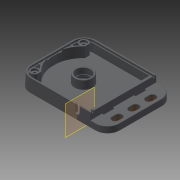
# Autodesk Inventor part: 276-2156
Saved by Autodesk Inventor 2016 SP2 (Build 200236200, 236)
## iProperties
Category: Sensors
Company: Autodesk Inc.
Created: 2012-04-02
Part Number: 276-2156
Document SubType Name: Modeling
Designer: Autodesk Inc.
Density: 1.42 g/cm^3
Material: Acetal Resin, White
Catalog Web Link: http://www.vexrobotics.com/276-2156.html
Vendor: VEX
Mass: 13.8512 g
Surface Area: 116.5 cm^2
Volume: 9.75434 cm^3
Appearance: Gray
Author: Autodesk Inc.
Autodesk Inventor part; units mm, degrees
(part 1 of 3)
sketch "Sketch1" plane through (0, 0, 0) normal (0, 0, 1) x (1, 0, 0)
  line L0 (61.4848, -6.4998) -> (61.4848, 43.5002)
  line L1 (53.0765, 43.5002) -> (-6.0152, 43.5002)
  line L2 (-6.0152, 43.5002) -> (-6.0152, -6.4998)
  line L3 (-6.0152, 43.5002) -> (61.4848, 43.5002)
  line L4 (-6.0152, -6.4998) -> (61.4848, -6.4998)
  constraints: 10 end point, 1 parallel
extrude "Extrusion1" add sketch "Sketch1" against normal blind 9.4996 draft -2
ref_plane "Work Plane1" through (-6.0152, -6.4998, 0) normal (0, 1, 0) x (1, 0, 0)
sketch "Sketch2" plane through (-6.0152, -6.4998, 0) normal (0, 1, 0) x (1, 0, 0)
  line L0 (0.3317, 9.4996) -> (67.1683, 9.4996)
  line L1 (67.5, 0) -> (67.1683, 9.4996)
  line L2 (0, 0) -> (67.5, 0)
  line L3 (0, 0) -> (0.3317, 9.4996)
  line L4 (0.157, 4.4958) -> (13.081, 4.4958)
  line L5 (13.081, 4.4958) -> (13.1683, 9.4996)
  point P0 (6.0152, 0)
  dimension "d3" = 5.0038
  dimension "d4" = 91
  dimension "d5" = 13.081
  constraints: 4 end point, 2 point on line, 1 parallel
  measures "d3" distance between parallel lines of L0 L4
  measures "d4" angle of L5 L4
  measures "d5" horizontal distance of L4.end L2.start
extrude "Extrusion2" cut sketch "Sketch2" along normal up to next contours L0 L5 L4 L3
fillet "Fillet1" radius 8.9916 4 edges at (61.3189, -6.3339, -4.7498) (-5.9367, -6.4213, -2.2479) (-5.9367, 43.4217, -2.2479) (61.3189, 43.3344, -4.7498)
ref_plane "Work Plane2" through (0, 0, -8.001) normal (0, 0, -1) x (-1, 0, 0)
sketch "Sketch5" plane through (0, 0, -9.4996) normal (0, 0, -1) x (-1, 0, 0)
  line L0 (-7.1531, -6.168) -> (-7.1531, 43.1685)
  line L1 (-52.1669, 43.1685) -> (-7.1531, 43.1685)
  arc A0 (-60.1554, 2.5074) -> (-52.4976, -5.1612) centre (-52.4864, 2.5078) ccw
  line L2 (-60.1554, 2.5074) -> (-60.1554, 34.509)
  arc A1 (-52.4904, 42.1754) -> (-60.1554, 34.509) centre (-52.4891, 34.509) ccw
  line L3 (-52.4904, 42.1754) -> (-7.6488, 42.1754)
  line L4 (-7.6488, 43.1685) -> (-52.4917, 43.1685)
  arc A2 (-52.4917, 43.1685) -> (-61.1599, 34.5002) centre (-52.4917, 34.5002) ccw
  line L5 (-18.6416, -6.168) -> (-52.4917, -6.168)
  ellipse E0 centre (-18.6417, -5.8678) end of major axis (-18.5647, -6.158) minor radius 0.3 (-18.6416, -6.168) -> (-18.3417, -5.8679) ccw
  line L6 (-18.3417, -5.8679) -> (-18.3417, -5.1612)
  line L7 (-7.1313, -5.1612) -> (-52.4976, -5.1612)
  arc A3 (-59.5458, 2.5026) -> (-52.4917, -4.5516) centre (-52.4917, 2.5026) ccw
  line L8 (-59.5458, 2.5026) -> (-59.5458, 5.6742)
  line L9 (-59.5458, 2.5026) -> (-59.5458, 34.5071)
  arc A4 (-52.4917, 41.5612) -> (-59.5458, 34.5071) centre (-52.4917, 34.5071) ccw
  line L10 (-8.9376, 41.5612) -> (-8.9376, -3.8612)
  line L11 (-8.9376, 40.8754) -> (-7.1313, 40.8754)
  line L12 (-7.1313, 40.8754) -> (-7.1313, 42.1832)
  line L13 (-7.1313, 42.1832) -> (-52.4904, 42.1754)
  arc A5 (-52.4904, 42.1754) -> (-60.1586, 34.5071) centre (-52.4904, 34.5071) ccw
  line L14 (-60.1586, 34.5071) -> (-60.1599, 2.5071)
  arc A6 (-60.1599, 2.5071) -> (-52.4917, -5.1612) centre (-52.4917, 2.5071) ccw
  line L15 (-52.4917, -5.1612) -> (-18.3278, -5.1612)
  line L16 (-8.9376, -4.5516) -> (-52.4917, -4.5516)
  line L17 (-8.9376, -3.8612) -> (-8.9376, -4.5516)
  line L18 (-8.9376, -3.8612) -> (-7.1313, -3.8612)
  line L19 (-7.1313, -3.8612) -> (-7.1313, -5.1612)
  line L20 (-52.4917, 41.5612) -> (-8.9376, 41.5612)
  line L21 (-7.1531, -6.168) -> (-52.1669, -6.168)
  line L22 (-8.9376, 41.5612) -> (-52.4917, 41.5612)
  arc A7 (-52.4917, 41.5612) -> (-59.5458, 34.5071) centre (-52.4917, 34.5071) ccw
  line L23 (-59.5458, 34.5071) -> (-59.5458, 2.5026)
  arc A8 (-59.5458, 2.5026) -> (-52.4917, -4.5516) centre (-52.4917, 2.5026) ccw
  line L24 (-52.4917, -4.5516) -> (-8.9376, -4.5516)
  line L25 (-8.9376, -4.5516) -> (-8.9376, 41.5612)
  point P0 (0, 0)
  point P1 (-6.9917, 18.5071)
  point P2 (-52.4917, 34.5071)
  dimension "d10" = 8.6614
  dimension "d13" = 0.9931
  dimension "d14" = 0.6096
  dimension "d15" = 0.6096
  dimension "d16" = 7.0541
  dimension "d17" = 7.6682
  dimension "d18" = 8.6683
  dimension "d19" = 7.0541
  constraints: 46 end point, 20 point on circle, 14 tangent, 9 centre point, 6 collinear, 5 perpendicular, 3 parallel, 3 vertical, 2 horizontal, 2 point on line, 5 other
  measures "d10" distance from line of point (-52.492, 34.507) L1
  measures "d13" distance between parallel lines of L3 L4
  measures "d14" distance between parallel lines of L16 L15
  measures "d15" distance between parallel lines of L2 L9
  measures "d16" radius of A4
  measures "d17" radius of A5
  measures "d18" radius of A2
  measures "d19" radius of A3
extrude "Extrusion3" cut sketch "Sketch5" against normal blind 1.4986 contours L7 A0 L2 A1 L13 L0 L11 L10 L20 A4 L9 L8 A3 L16 L17 L18 | L0 L18 L19 L7 | L0 L13 L12 L11 | L17 L16 A3 L8 L9 A4 L20 L10
extrude "Extrusion4" cut sketch "Sketch5" against normal blind 6.1976 draft -0.5 contours L17 L16 A3 L8 L9 A4 L20 L10
sketch "Sketch9" plane through (0, 0, 0) normal (0, 0, 1) x (1, 0, 0)
  circle A0 centre (37.0754, 18.4938) radius 4.7498
  circle A1 centre (37.0754, 18.4938) radius 5.3086
  point P0 (0, 0)
  dimension "d36" = 10.6172
  constraints: 1 centre point, 1 coincident
  measures "d36" diameter of A1
sketch "Sketch10" plane through (0, 0, -9.4996) normal (0, 0, -1) x (-1, 0, 0)
  circle A0 centre (-37.0754, 18.4938) radius 4.7498
  arc A1 (-56.912, 5.8938) -> (-52.4754, 0.7431) centre (-37.0754, 18.4938) ccw
  line L0 (-52.4754, 0.7431) -> (-52.4754, 1.9978)
  arc A2 (-59.5458, 16.4056) -> (-52.4754, 1.9978) centre (-37.0754, 18.4938) ccw
  line L1 (-58.9436, 12.9209) -> (-58.9436, 9.8898)
  arc A3 (-60.1436, 14.0099) -> (-57.6251, 7.0938) centre (-37.0754, 18.4938) ccw
  line L2 (-57.6251, 7.0938) -> (-60.1436, 7.0938)
  line L3 (-58.9436, 7.0938) -> (-58.9436, 5.8938)
  line L4 (-60.1436, 5.8938) -> (-56.912, 5.8938)
  line L5 (-58.9436, 7.0938) -> (-57.6251, 7.0938)
  arc A4 (-58.9436, 9.8898) -> (-57.6251, 7.0938) centre (-37.0754, 18.4938) ccw
  line L6 (-58.9436, 9.8898) -> (-58.9436, 12.9209)
  arc A5 (-58.9436, 12.9209) -> (-52.4754, 1.9978) centre (-37.0754, 18.4938) ccw
  line L7 (-52.4754, 1.9978) -> (-52.4754, 0.7431)
  arc A6 (-56.912, 5.8938) -> (-52.4754, 0.7431) centre (-37.0754, 18.4938) ccw
  line L8 (-56.912, 5.8938) -> (-58.9436, 5.8938)
  line L9 (-58.9436, 5.8938) -> (-58.9436, 7.0938)
  line L10 (-57.6251, 29.8938) -> (-60.1436, 29.8938)
  line L11 (-58.9436, 29.8938) -> (-58.9436, 31.0938)
  line L12 (-60.1436, 31.0938) -> (-56.912, 31.0938)
  arc A7 (-52.4754, 36.2446) -> (-56.912, 31.0938) centre (-37.0754, 18.4938) ccw
  line L13 (-52.4754, 36.2446) -> (-52.4754, 34.9898)
  arc A8 (-52.4754, 34.9898) -> (-59.5458, 20.5821) centre (-37.0754, 18.4938) ccw
  line L14 (-58.9436, 24.0668) -> (-58.9436, 27.0979)
  arc A9 (-57.6251, 29.8938) -> (-60.1436, 22.9778) centre (-37.0754, 18.4938) ccw
  arc A10 (-52.4754, 42.1621) -> (-60.1436, 34.4938) centre (-52.4754, 34.4938) ccw
  line L15 (-60.1436, 34.4938) -> (-60.1436, 2.4938)
  arc A11 (-60.1436, 2.4938) -> (-52.4754, -5.1744) centre (-52.4754, 2.4938) ccw
  arc A12 (-61.1436, 2.4938) -> (-52.4754, -6.1744) centre (-52.4754, 2.4938) ccw
  line L16 (-61.1436, 2.4938) -> (-61.1436, 34.4938)
  arc A13 (-52.4754, 43.1621) -> (-61.1436, 34.4938) centre (-52.4754, 34.4938) ccw
  arc A14 (-57.0545, -2.8468) -> (-52.4754, -1.2562) centre (-55.4754, -0.0062) ccw
  line L17 (-52.4754, -1.2562) -> (-52.4754, 0.7431)
  arc A15 (-54.9133, 3.1949) -> (-52.4754, 0.7431) centre (-37.0754, 18.4938) ccw
  arc A16 (-54.9133, 3.1949) -> (-58.5542, -1.0471) centre (-55.4754, -0.0062) ccw
  arc A17 (-58.5542, -1.0471) -> (-57.0545, -2.8468) centre (-52.4754, 2.4938) ccw
  circle A18 centre (-55.4754, -0.0062) radius 2.2762
  arc A19 (-52.4754, 36.2446) -> (-54.9133, 33.7928) centre (-37.0754, 18.4938) ccw
  line L18 (-52.4754, 36.2446) -> (-52.4754, 38.2438)
  arc A20 (-52.4754, 38.2438) -> (-57.0545, 39.8344) centre (-55.4754, 36.9938) ccw
  arc A21 (-57.0545, 39.8344) -> (-58.5542, 38.0348) centre (-52.4754, 34.4938) ccw
  arc A22 (-58.5542, 38.0348) -> (-54.9133, 33.7928) centre (-55.4754, 36.9938) ccw
  circle A23 centre (-55.4754, 36.9938) radius 2.2762
  line L19 (-59.5458, 2.5026) -> (-59.5458, 34.5071)
  point P0 (0, 0)
  constraints: 46 point on circle, 38 end point, 23 centre point, 12 point on line
extrude "Extrusion10" add sketch "Sketch10" against normal up to surface (6.1976 mm away) contours L4 L3 L2 A3 L1 A2 L0 A1 | L4 L19 L2 L3 | L4 L15 L2 L19 | L1 A3 L19 A2 | A3 L15 A9 L19 | L19 A9 L14 A8 | L14 A9 L10 L11 L12 A7 L13 A8 | L15 L12 L19 L10 | L19 L12 L11 L10
sketch "Sketch11" plane through (0, 0, -9.4996) normal (0, 0, -1) x (-1, 0, 0)
  line L0 (-60.1554, 2.5074) -> (-60.1554, 34.509)
  line L1 (-60.1554, 5.8904) -> (-60.1554, 7.1091)
  line L2 (-59.5458, 2.5026) -> (-59.5458, 34.5071)
  line L3 (-60.1436, 34.4938) -> (-60.1436, 2.4938)
  line L4 (-59.5458, 29.8998) -> (-60.1436, 29.8998)
  line L5 (-60.1436, 29.8998) -> (-60.1436, 31.0963)
  line L6 (-60.1436, 31.0963) -> (-59.5458, 31.0963)
  line L7 (-59.5458, 31.0963) -> (-59.5458, 29.8998)
  line L8 (-60.1436, 5.8938) -> (-56.912, 5.8938)
  line L9 (-59.5458, 5.8938) -> (-60.1436, 5.8938)
  line L10 (-60.1436, 5.8938) -> (-60.1436, 7.0942)
  line L11 (-60.1436, 7.0942) -> (-59.5458, 7.0942)
  line L12 (-59.5458, 7.0942) -> (-59.5458, 5.8938)
  line L13 (-58.9436, 9.8898) -> (-58.9436, 12.9209)
  arc A0 (-60.1436, 14.0099) -> (-57.6251, 7.0938) centre (-37.0754, 18.4938) ccw
  arc A1 (-57.6251, 29.8938) -> (-60.1436, 22.9778) centre (-37.0754, 18.4938) ccw
  line L14 (-58.9436, 24.0668) -> (-58.9436, 27.0979)
  arc A2 (-52.4754, 34.9898) -> (-59.5458, 20.5821) centre (-37.0754, 18.4938) ccw
  line L15 (-59.5458, 16.4056) -> (-59.5458, 20.5821)
  arc A3 (-59.5458, 16.4056) -> (-52.4754, 1.9978) centre (-37.0754, 18.4938) ccw
  point P0 (0, 0)
  constraints: 18 end point, 6 point on line, 4 parallel, 2 horizontal, 2 perpendicular
extrude "Extrusion11" cut sketch "Sketch11" against normal up to surface (1.4986 mm away) contours L8 L3 L11 L2 | A0 L3 A1 L2 | L2 A3 L13 A0 | L2 A1 L14 A2 | L3 L6 L2 L4
extrude "Extrusion12" add sketch "Sketch10" against normal up to surface (6.1976 mm away) contours A1 L17 A14 A17 A16 | A7 A22 A21 A20 L18 | A18 | A23
extrude "Extrusion13" cut sketch "Sketch10" against normal blind 1.4986 contours A18 | A23
hole "Hole1" at (55.4754, -0.0062, -9.4996) at (55.4754, 36.9938, -9.4996) direction (0, 0, 1) diameter 2.1082 end through all
ref_plane "Work Plane3" through (27.7348, -6.4998, 0) normal (0, 1, 0) x (-1, 0, 0)
sketch "Sketch12" plane through (27.7348, -6.4998, 0) normal (0, 1, 0) x (-1, 0, 0)
  line L0 (24.7639, 0) -> (-24.7639, 0)
  line L1 (9.4422, -3.81) -> (12.0584, -3.81)
  line L2 (12.0584, -3.81) -> (12.116, -9.4996)
  line L3 (9.4422, -3.81) -> (9.3846, -9.4996)
  line L4 (20.5817, -9.4996) -> (-24.4321, -9.4996)
  point P0 (27.7348, 0)
  point P1 (20.669, -4.4958)
  dimension "d59" = 3.81
  dimension "d60" = 8.6106
  dimension "d61" = 90.58
  dimension "d62" = 90.58
  dimension "d63" = 2.6162
  constraints: 6 end point, 2 point on line, 1 parallel
  measures "d59" distance between parallel lines of L1 L0
  measures "d60" horizontal distance of L1.end point (20.669, -4.496)
  measures "d61" angle of L2 L1
  measures "d62" angle of L3 L1
  measures "d63" distance of L1.start L1.end
extrude "Extrusion14" cut sketch "Sketch12" along normal up to next
fillet "Fillet6" radius 0.508 5 edges at (18.3214, -6.2674, -6.6548) (16.9845, -6.3667, -3.81) (15.6476, -6.2674, -6.6548) (18.2926, -5.4343, -3.81) (15.6764, -5.4343, -3.81)
extrude "Extrusion15" cut sketch "Sketch10" against normal up to surface (1.4986 mm away) contours L4 L19 L2 L3 | L4 L15 L2 L19 | L15 L12 L19 L10 | L19 L12 L11 L10
sketch "Sketch13" plane through (0, 0, 0) normal (0, 0, 1) x (1, 0, 0)
  line L0 (52.4987, 43.5002) -> (2.9709, 43.5002)
  line L1 (-6.0152, 34.5141) -> (-6.0152, 2.4864)
  line L2 (2.9709, -6.4998) -> (52.4987, -6.4998)
  point P0 (0, 0)
  point P1 (12.0442, 36.9978)
  point P2 (12.0442, 0.0026)
  dimension "d69" = 6.5024
  dimension "d70" = 18.0594
  dimension "d71" = 6.5024
  constraints: 1 vertical alignment
  measures "d69" distance from line of L0 point (12.044, 36.998)
  measures "d70" distance from line of L1 point (12.044, 36.998)
  measures "d71" distance from line of L2 point (12.044, 0.003)
hole "Hole2" at (12.0442, 36.9978, 0) at (12.0442, 0.0026, 0) direction (0, 0, -1) diameter 3.7846 depth 3.302
fillet "Fillet7" radius 0.508 2 edges at (12.0442, 1.8949, 0) (12.0442, 38.8901, 0)
sketch "Sketch14" plane through (7.0658, -6.3428, -4.4958) normal (0, 0, -1) x (-1, 0, 0)
  arc A0 (1.2904, 16.6628) -> (1.0904, 16.8628) centre (1.0904, 16.6628) ccw
  line L0 (1.2904, 16.6628) -> (1.2904, 9.0104)
  arc A1 (1.0904, 8.8104) -> (1.2904, 9.0104) centre (1.0904, 9.0104) ccw
  line L1 (1.0904, 8.8104) -> (0.2119, 8.8104)
  ellipse E0 centre (0.2119, 9.0104) end of major axis (0.3908, 9.0999) minor radius 0.2 (0.0119, 9.0104) -> (0.2119, 8.8104) ccw
  line L2 (3.9556, 0.4766) -> (0.0119, 0.4766)
  ellipse E1 centre (3.9461, 8.9809) end of major axis (-2.0703, 14.9981) minor radius 8.4995 (3.9556, 0.4766) -> (12.4504, 8.9714) ccw
  line L3 (12.4504, 40.7018) -> (12.4504, 8.9714)
  ellipse E2 centre (3.9461, 40.6923) end of major axis (9.9626, 46.7095) minor radius 8.4995 (12.4504, 40.7018) -> (3.9556, 49.1966) ccw
  ellipse E3 centre (0.2121, 40.6628) end of major axis (0.0332, 40.7522) minor radius 0.2 (0.2121, 40.8628) -> (0.0121, 40.6628) ccw
  line L4 (1.0907, 40.8628) -> (0.2121, 40.8628)
  arc A2 (1.2904, 40.6628) -> (1.0907, 40.8628) centre (1.0904, 40.6628) ccw
  line L5 (1.2904, 40.6628) -> (1.2904, 33.0104)
  arc A3 (1.0904, 32.8104) -> (1.2904, 33.0104) centre (1.0904, 33.0104) ccw
  line L6 (1.0904, 32.8104) -> (0.2119, 32.8104)
  ellipse E4 centre (0.2119, 33.0104) end of major axis (0.3908, 33.0999) minor radius 0.2 (0.0119, 33.0104) -> (0.2119, 32.8104) ccw
  ellipse E5 centre (0.2119, 16.6628) end of major axis (0.033, 16.7522) minor radius 0.2 (0.2119, 16.8628) -> (0.0119, 16.6628) ccw
  line L7 (1.0904, 16.8628) -> (0.2119, 16.8628)
  arc A4 (10.8404, 26.3366) -> (5.3404, 26.3366) centre (8.0904, 26.3366) ccw
  line L8 (10.8404, 23.3366) -> (10.8404, 26.3366)
  arc A5 (5.3404, 23.3366) -> (10.8404, 23.3366) centre (8.0904, 23.3366) ccw
  line L9 (5.3404, 26.3366) -> (5.3404, 23.3366)
  arc A6 (10.8404, 39.0366) -> (5.3404, 39.0366) centre (8.0904, 39.0366) ccw
  line L10 (10.8404, 36.0366) -> (10.8404, 39.0366)
  arc A7 (5.3404, 36.0366) -> (10.8404, 36.0366) centre (8.0904, 36.0366) ccw
  line L11 (5.3404, 39.0366) -> (5.3404, 36.0366)
  arc A8 (10.8404, 13.6366) -> (5.3404, 13.6366) centre (8.0904, 13.6366) ccw
  line L12 (10.8404, 10.6366) -> (10.8404, 13.6366)
  arc A9 (5.3404, 10.6366) -> (10.8404, 10.6366) centre (8.0904, 10.6366) ccw
  line L13 (5.3404, 13.6366) -> (5.3404, 10.6366)
  line L14 (0.0119, 9.0104) -> (0.0119, 16.6628)
  line L15 (0.0121, 33.0005) -> (0.0121, 40.6628)
  point P0 (7.0658, 6.3428)
  point P1 (0.0904, 24.8366)
  point P2 (-30.0215, 24.36)
  point P3 (-30.0096, 24.8366)
  constraints: 32 end point, 20 point on circle, 10 centre point, 2 parallel, 28 other
extrude "Extrusion17" cut sketch "Sketch14" against normal blind 2.9972 contours L0 A1 L1 E0 L14 E5 L7 A0 | L4 A2 L5 A3 L6 E4 L15 E3
sketch "Sketch18" plane through (0, 0, -3.302) normal (0, 0, -1) x (-1, 0, 0)
  circle A0 centre (-12.0442, 0.0026) radius 1.8923
  circle A1 centre (-12.0442, 36.9978) radius 1.8923
  arc A2 (-56.9239, -2.9155) -> (-52.4754, -1.2562) centre (-55.4754, -0.0062) ccw
  arc A3 (-56.9239, -2.9155) -> (-52.4917, -4.4975) centre (-52.4917, 2.5026) ccw
  line L0 (-52.4917, -4.4975) -> (-8.9916, -4.4975)
  line L1 (-8.9916, -4.4975) -> (-8.9916, 41.5071)
  line L2 (-8.9916, 41.5071) -> (-52.4917, 41.5071)
  arc A4 (-52.4917, 41.5071) -> (-56.9935, 39.8675) centre (-52.4917, 34.5071) ccw
  arc A5 (-52.4754, 38.2438) -> (-56.9935, 39.8675) centre (-55.4754, 36.9938) ccw
  line L3 (-52.4754, 38.2438) -> (-52.4754, 34.9898)
  arc A6 (-52.4754, 34.9898) -> (-59.4917, 21.0993) centre (-37.0754, 18.4938) ccw
  line L4 (-59.4917, 21.0993) -> (-59.4917, 15.8884)
  arc A7 (-59.4917, 15.8884) -> (-52.4754, 1.9978) centre (-37.0754, 18.4938) ccw
  line L5 (-52.4754, 1.9978) -> (-52.4754, -1.2562)
  circle A8 centre (-37.0754, 18.4938) radius 7.2429
  point P0 (0, 0)
extrude "Extrusion20" cut sketch "Sketch18" against normal blind 1.4986 contours A2 L5 A7 L4 A6 L3 A5 A4 L2 L1 L0 A3 | A8
sketch "Sketch19" plane through (0, 0, -1.8034) normal (0, 0, -1) x (-1, 0, 0)
  arc A0 (-59.4917, 15.8884) -> (-52.4754, 1.9978) centre (-37.0754, 18.4938) ccw
  circle A1 centre (-37.0754, 18.4938) radius 6.7437
  point P0 (-37.0754, 18.4938)
  point P1 (0, 0)
  dimension "d92" = 13.4874
  constraints: 1 centre point, 1 coincident
  measures "d92" diameter of A1
extrude "Extrusion21" add sketch "Sketch19" along normal blind 6.2484 draft -1
sketch "Sketch20" plane through (37.0754, 18.4938, -8.0518) normal (0, 0, -1) x (-1, 0, 0)
  circle A0 centre (0, 0) radius 6.6346
  circle A1 centre (0, 0) radius 5.2451
  point P0 (37.0754, -18.4938)
  dimension "d95" = 10.4902
  constraints: 1 centre point, 1 coincident
  measures "d95" diameter of A1
extrude "Extrusion22" cut sketch "Sketch20" against normal blind 4.5466 contours A1
sketch "Sketch21" plane through (37.0754, 18.4938, -3.5052) normal (0, 0, -1) x (-1, 0, 0)
  circle A0 centre (0, 0) radius 5.2451
  circle A1 centre (0, 0) radius 4.7498
  point P0 (37.0754, -18.4938)
  dimension "d98" = 9.4996
  constraints: 1 centre point, 1 coincident
  measures "d98" diameter of A1
extrude "Extrusion23" cut sketch "Sketch21" against normal through all contours A1
extrude "Extrusion24" cut sketch "Sketch9" against normal blind 2.159
fillet "Fillet10" radius 1.4986 1 edges at (31.7668, 18.4938, 0)
fillet "Fillet11" radius 0.508 2 edges at (31.7668, 18.4938, -2.159) (41.8252, 18.4938, -2.159)
fillet "Fillet12" radius 0.508 2 edges at (43.71, 18.4938, -8.0518) (42.3205, 18.4938, -8.0518)
sketch "Sketch22" plane through (0, 0, 0) normal (0, 0, 1) x (1, 0, 0)
  line L0 (-6.004, 2.4925) -> (-6.004, 34.5035)
  line L1 (-6.004, 34.5035) -> (-6.004, 2.4925)
  ellipse E0 centre (-4.7038, 16.343) end of major axis (-4.4914, 16.5554) minor radius 0.3 (-5.004, 16.3427) -> (-4.7042, 16.0429) ccw
  spline S0 degree 3 poles (-5.379, 16.1568) (-5.3713, 16.112) (-5.3586, 16.0685) (-5.3265, 15.991) (-5.3082, 15.9569) (-5.2649, 15.8923) (-5.2385, 15.8606) (-5.1846, 15.8064) (-5.155, 15.7821) (-5.0906, 15.7392) (-5.0541, 15.7199) (-4.9466, 15.6745) (-4.8699, 15.6592) (-4.7883, 15.6589) knots 0.106772 0.106772 0.106772 0.106772 0.25 0.25 0.375 0.375 0.5 0.5 0.625 0.625 0.75 0.75 1 1 1 1
  spline S1 degree 3 poles (-5.388, 16.2585) (-5.3876, 16.1781) (-5.3714, 16.0993) (-5.3265, 15.991) (-5.3082, 15.9569) (-5.2649, 15.8923) (-5.2385, 15.8606) (-5.1846, 15.8064) (-5.155, 15.7821) (-5.0906, 15.7392) (-5.0541, 15.7199) (-4.9466, 15.6745) (-4.8699, 15.6592) (-4.7883, 15.6589) knots 0 0 0 0 0.25 0.25 0.375 0.375 0.5 0.5 0.625 0.625 0.75 0.75 1 1 1 1
  spline S2 degree 3 poles (-5.388, 16.2585) (-5.3878, 16.2242) (-5.3848, 16.1901) (-5.379, 16.1568) knots 0 0 0 0 1 1 1 1
  spline S3 degree 3 poles (-5.379, 16.1568) (-5.3755, 16.1426) (-5.3722, 16.1319) (-5.3702, 16.1262) (-5.3698, 16.1252) (-5.3695, 16.1244) (-5.3694, 16.1244) (-5.3693, 16.124) (-5.3691, 16.1237) (-5.369, 16.1236) (-5.369, 16.1235) (-5.369, 16.1235) (-5.369, 16.1235) (-5.3689, 16.1235) (-5.3689, 16.1235) (-5.3689, 16.1235) (-5.3689, 16.1235) (-5.3689, 16.1235) (-5.3689, 16.1235) (-5.3689, 16.1235) (-5.3689, 16.1235) (-5.3689, 16.1236) (-5.3689, 16.1236) (-5.3689, 16.1237) (-5.3689, 16.1238) (-5.369, 16.125) (-5.3696, 16.1282) (-5.3755, 16.1555) (-5.3847, 16.1961) (-5.388, 16.2585) knots 0 0 0 0 0.216458 0.216458 0.250147 0.250147 0.25213 0.25213 0.266562 0.266562 0.270758 0.270758 0.271952 0.271952 0.272738 0.272738 0.27341 0.27341 0.274154 0.274154 0.275352 0.275352 0.277883 0.277883 0.289351 0.289351 0.40678 0.40678 1 1 1 1
  spline S4 degree 3 poles (-1.886, 13.7062) (-2.182, 13.7856) (-2.4626, 13.9029) (-2.7267, 14.0575) (-2.9908, 14.2122) (-3.23, 14.3994) (-3.4442, 14.6191) knots 0 0 0 0 0.5 0.5 0.5 1 1 1 1
  spline S5 degree 3 poles (-1.886, 13.7062) (-2.182, 13.7856) (-2.4626, 13.9029) (-2.7267, 14.0575) (-2.9908, 14.2122) (-3.23, 14.3994) (-3.4442, 14.6191) knots 0 0 0 0 0.5 0.5 0.5 1 1 1 1
  arc A0 (-3.7192, 14.351) -> (-1.9854, 13.3353) centre (-1.004, 16.998) ccw
  line L2 (-4.5461, 14.1709) -> (-4.5461, 10.1251)
  line L3 (-4.5461, 14.1709) -> (-4.5461, 10.1251)
  line L4 (-4.1621, 10.1251) -> (-4.1621, 14.1709)
  line L5 (2.4039, 17.398) -> (2.4039, 16.998)
  line L6 (2.7879, 16.998) -> (2.7879, 17.398)
  spline S6 degree 3 poles (3.246, 18.2401) (3.1925, 18.24) (3.1399, 18.2351) (3.0882, 18.2252) (3.0624, 18.2203) (3.0368, 18.2142) (3.0114, 18.2068) (2.9861, 18.1994) (2.963, 18.1916) (2.936, 18.1809) (2.8282, 18.1383) (2.7326, 18.0753) (2.6506, 17.9934) (2.6096, 17.9525) (2.5734, 17.9082) (2.5422, 17.8606) (2.5266, 17.8368) (2.5121, 17.8122) (2.499, 17.7868) (2.4924, 17.774) (2.4861, 17.7611) (2.4801, 17.748) (2.4741, 17.7348) (2.468, 17.7203) (2.4631, 17.7079) (2.4237, 17.6087) (2.404, 17.5054) (2.4039, 17.398) knots 0 0 0 0 0.125 0.125 0.125 0.1875 0.1875 0.1875 0.25 0.25 0.25 0.5 0.5 0.5 0.625 0.625 0.625 0.6875 0.6875 0.6875 0.71875 0.71875 0.71875 0.75 0.75 0.75 1 1 1 1
  spline S7 degree 3 poles (3.246, 18.2401) (3.1925, 18.24) (3.1399, 18.2351) (3.0882, 18.2252) (3.0624, 18.2203) (3.0368, 18.2142) (3.0114, 18.2068) (2.9861, 18.1994) (2.963, 18.1916) (2.936, 18.1809) (2.8282, 18.1383) (2.7326, 18.0753) (2.6506, 17.9934) (2.6096, 17.9525) (2.5734, 17.9082) (2.5422, 17.8606) (2.5266, 17.8368) (2.5121, 17.8122) (2.499, 17.7868) (2.4924, 17.774) (2.4861, 17.7611) (2.4801, 17.748) (2.4741, 17.7348) (2.468, 17.7203) (2.4631, 17.7079) (2.4237, 17.6087) (2.404, 17.5054) (2.4039, 17.398) knots 0 0 0 0 0.125 0.125 0.125 0.1875 0.1875 0.1875 0.25 0.25 0.25 0.5 0.5 0.5 0.625 0.625 0.625 0.6875 0.6875 0.6875 0.71875 0.71875 0.71875 0.75 0.75 0.75 1 1 1 1
  arc A1 (3.246, 17.8561) -> (2.7879, 17.398) centre (3.246, 17.398) ccw
  line L7 (6.996, 17.8561) -> (3.246, 17.8561)
  line L8 (6.996, 18.2401) -> (3.246, 18.2401)
  line L9 (6.996, 18.2401) -> (3.246, 18.2401)
  line L10 (7.4541, 17.398) -> (7.4541, 12.498)
  line L11 (7.8381, 12.498) -> (7.8381, 17.398)
  line L12 (7.8381, 12.498) -> (7.8381, 17.398)
  arc A2 (7.4541, 17.398) -> (6.996, 17.8561) centre (6.996, 17.398) ccw
  spline S8 degree 3 poles (7.8381, 17.398) (7.8381, 17.4515) (7.833, 17.5041) (7.8232, 17.5558) (7.8182, 17.5816) (7.8121, 17.6072) (7.8048, 17.6326) (7.7974, 17.6579) (7.7896, 17.681) (7.779, 17.7079) (7.7363, 17.8157) (7.6734, 17.9114) (7.5914, 17.9934) (7.5505, 18.0344) (7.5061, 18.0704) (7.4585, 18.1017) (7.4229, 18.1251) (7.3854, 18.1459) (7.346, 18.1639) (7.3329, 18.1699) (7.3184, 18.176) (7.306, 18.1809) (7.2067, 18.2202) (7.1034, 18.24) (6.996, 18.2401) knots 0 0 0 0 0.125 0.125 0.125 0.1875 0.1875 0.1875 0.25 0.25 0.25 0.5 0.5 0.5 0.625 0.625 0.625 0.71875 0.71875 0.71875 0.75 0.75 0.75 1 1 1 1
  spline S9 degree 3 poles (7.8381, 17.398) (7.8381, 17.4515) (7.833, 17.5041) (7.8232, 17.5558) (7.8182, 17.5816) (7.8121, 17.6072) (7.8048, 17.6326) (7.7974, 17.6579) (7.7896, 17.681) (7.779, 17.7079) (7.7363, 17.8157) (7.6734, 17.9114) (7.5914, 17.9934) (7.5505, 18.0344) (7.5061, 18.0704) (7.4585, 18.1017) (7.4229, 18.1251) (7.3854, 18.1459) (7.346, 18.1639) (7.3329, 18.1699) (7.3184, 18.176) (7.306, 18.1809) (7.2067, 18.2202) (7.1034, 18.24) (6.996, 18.2401) knots 0 0 0 0 0.125 0.125 0.125 0.1875 0.1875 0.1875 0.25 0.25 0.25 0.5 0.5 0.5 0.625 0.625 0.625 0.71875 0.71875 0.71875 0.75 0.75 0.75 1 1 1 1
  line L13 (2.4039, 17.398) -> (2.4039, 16.998)
  spline S10 degree 3 poles (-3.87, 8.0375) (-3.8702, 8.0718) (-3.8732, 8.1058) (-3.879, 8.1392) knots 0 0 0 0 1 1 1 1
  spline S11 degree 3 poles (-3.879, 8.1392) (-3.8825, 8.1533) (-3.8858, 8.164) (-3.8878, 8.1697) (-3.8882, 8.1708) (-3.8885, 8.1716) (-3.8885, 8.1716) (-3.8887, 8.172) (-3.8888, 8.1722) (-3.889, 8.1724) (-3.889, 8.1724) (-3.889, 8.1725) (-3.889, 8.1725) (-3.889, 8.1725) (-3.889, 8.1725) (-3.889, 8.1725) (-3.8891, 8.1725) (-3.8891, 8.1725) (-3.8891, 8.1724) (-3.8891, 8.1724) (-3.8891, 8.1724) (-3.8891, 8.1724) (-3.8891, 8.1724) (-3.8891, 8.1723) (-3.8891, 8.1722) (-3.889, 8.171) (-3.8883, 8.1678) (-3.8824, 8.1405) (-3.8733, 8.0998) (-3.87, 8.0375) knots 0 0 0 0 0.216458 0.216458 0.250147 0.250147 0.25213 0.25213 0.266562 0.266562 0.270758 0.270758 0.271952 0.271952 0.272738 0.272738 0.27341 0.27341 0.274154 0.274154 0.275352 0.275352 0.277883 0.277883 0.289351 0.289351 0.40678 0.40678 1 1 1 1
  ellipse E1 centre (-4.5542, 7.9529) end of major axis (-4.3418, 8.1653) minor radius 0.3 (-4.254, 7.9533) -> (-4.5538, 8.2531) ccw
  line L14 (-4.7042, 8.2531) -> (-4.5538, 8.2531)
  ellipse E2 centre (-4.7038, 7.9529) end of major axis (-4.9162, 8.1653) minor radius 0.3 (-4.7042, 8.2531) -> (-5.004, 7.9533) ccw
  spline S12 degree 3 poles (-3.879, 8.1392) (-3.8867, 8.1839) (-3.8994, 8.2275) (-3.9315, 8.3049) (-3.9498, 8.3391) (-3.9931, 8.4036) (-4.0194, 8.4354) (-4.0734, 8.4896) (-4.103, 8.5138) (-4.1674, 8.5567) (-4.2038, 8.5761) (-4.3114, 8.6214) (-4.388, 8.6367) (-4.4696, 8.6371) knots 0.106772 0.106772 0.106772 0.106772 0.25 0.25 0.375 0.375 0.5 0.5 0.625 0.625 0.75 0.75 1 1 1 1
  spline S13 degree 3 poles (-3.87, 8.0375) (-3.8704, 8.1178) (-3.8866, 8.1966) (-3.9315, 8.3049) (-3.9498, 8.3391) (-3.9931, 8.4036) (-4.0194, 8.4354) (-4.0734, 8.4896) (-4.103, 8.5138) (-4.1674, 8.5567) (-4.2038, 8.5761) (-4.3114, 8.6214) (-4.388, 8.6367) (-4.4696, 8.6371) knots 0 0 0 0 0.25 0.25 0.375 0.375 0.5 0.5 0.625 0.625 0.75 0.75 1 1 1 1
  line L15 (-4.4696, 8.6371) -> (-4.7883, 8.6371)
  line L16 (-4.4696, 8.6371) -> (-4.7883, 8.6371)
  spline S14 degree 3 poles (-4.7883, 8.6371) (-4.8227, 8.6369) (-4.8567, 8.6339) (-4.8901, 8.6281) knots 0 0 0 0 1 1 1 1
  spline S15 degree 3 poles (-4.8901, 8.6281) (-4.9042, 8.6246) (-4.9149, 8.6213) (-4.9206, 8.6193) (-4.9217, 8.6189) (-4.9224, 8.6186) (-4.9225, 8.6185) (-4.9229, 8.6184) (-4.9231, 8.6183) (-4.9233, 8.6181) (-4.9233, 8.6181) (-4.9233, 8.6181) (-4.9233, 8.6181) (-4.9233, 8.6181) (-4.9233, 8.6181) (-4.9233, 8.618) (-4.9233, 8.618) (-4.9233, 8.618) (-4.9233, 8.618) (-4.9233, 8.618) (-4.9233, 8.618) (-4.9233, 8.618) (-4.9233, 8.618) (-4.9232, 8.618) (-4.923, 8.618) (-4.9218, 8.6181) (-4.9186, 8.6188) (-4.8914, 8.6247) (-4.8507, 8.6338) (-4.7883, 8.6371) knots 0 0 0 0 0.216458 0.216458 0.250147 0.250147 0.25213 0.25213 0.266562 0.266562 0.270758 0.270758 0.271952 0.271952 0.272738 0.272738 0.27341 0.27341 0.274154 0.274154 0.275352 0.275352 0.277883 0.277883 0.289351 0.289351 0.40678 0.40678 1 1 1 1
  spline S16 degree 3 poles (-4.8901, 8.6281) (-4.9348, 8.6204) (-4.9784, 8.6077) (-5.0558, 8.5756) (-5.09, 8.5573) (-5.1545, 8.514) (-5.1862, 8.4877) (-5.2404, 8.4337) (-5.2647, 8.4041) (-5.3076, 8.3397) (-5.3269, 8.3032) (-5.3723, 8.1957) (-5.3876, 8.119) (-5.388, 8.0375) knots 0.106772 0.106772 0.106772 0.106772 0.25 0.25 0.375 0.375 0.5 0.5 0.625 0.625 0.75 0.75 1 1 1 1
  spline S17 degree 3 poles (-4.7883, 8.6371) (-4.8687, 8.6367) (-4.9475, 8.6205) (-5.0558, 8.5756) (-5.09, 8.5573) (-5.1545, 8.514) (-5.1862, 8.4877) (-5.2404, 8.4337) (-5.2647, 8.4041) (-5.3076, 8.3397) (-5.3269, 8.3032) (-5.3723, 8.1957) (-5.3876, 8.119) (-5.388, 8.0375) knots 0 0 0 0 0.25 0.25 0.375 0.375 0.5 0.5 0.625 0.625 0.75 0.75 1 1 1 1
  arc A3 (-3.254, 16.998) -> (1.246, 16.998) centre (-1.004, 16.998) ccw
  arc A4 (-3.254, 16.998) -> (1.246, 16.998) centre (-1.004, 16.998) ccw
  arc A5 (-0.0226, 13.3353) -> (2.7879, 16.998) centre (-1.004, 16.998) ccw
  spline S18 degree 3 poles (2.4039, 16.998) (2.4039, 16.8157) (2.3896, 16.6357) (2.3611, 16.458) (2.3468, 16.3691) (2.329, 16.2808) (2.3076, 16.1931) (2.2969, 16.1492) (2.2854, 16.1055) (2.2729, 16.0619) (2.2666, 16.0401) (2.2602, 16.0184) (2.2535, 15.9967) (2.2468, 15.975) (2.2403, 15.9545) (2.2328, 15.9316) (2.1123, 15.5657) (1.9342, 15.229) (1.6997, 14.9234) (1.5825, 14.7705) (1.4542, 14.6295) (1.3149, 14.5001) (1.2452, 14.4355) (1.1728, 14.3738) (1.0976, 14.315) (1.06, 14.2856) (1.0217, 14.257) (0.9828, 14.229) (0.9633, 14.2151) (0.9436, 14.2013) (0.9238, 14.1877) (0.904, 14.1741) (0.8828, 14.16) (0.8638, 14.1475) (0.5591, 13.9478) (0.2306, 13.8007) (-0.1219, 13.7062) knots 0 0 0 0 0.125 0.125 0.125 0.1875 0.1875 0.1875 0.21875 0.21875 0.21875 0.234375 0.234375 0.234375 0.25 0.25 0.25 0.5 0.5 0.5 0.625 0.625 0.625 0.6875 0.6875 0.6875 0.71875 0.71875 0.71875 0.734375 0.734375 0.734375 0.75 0.75 0.75 1 1 1 1
  spline S19 degree 3 poles (2.4039, 16.998) (2.4039, 16.8157) (2.3896, 16.6357) (2.3611, 16.458) (2.3468, 16.3691) (2.329, 16.2808) (2.3076, 16.1931) (2.2969, 16.1492) (2.2854, 16.1055) (2.2729, 16.0619) (2.2666, 16.0401) (2.2602, 16.0184) (2.2535, 15.9967) (2.2468, 15.975) (2.2403, 15.9545) (2.2328, 15.9316) (2.1123, 15.5657) (1.9342, 15.229) (1.6997, 14.9234) (1.5825, 14.7705) (1.4542, 14.6295) (1.3149, 14.5001) (1.2452, 14.4355) (1.1728, 14.3738) (1.0976, 14.315) (1.06, 14.2856) (1.0217, 14.257) (0.9828, 14.229) (0.9633, 14.2151) (0.9436, 14.2013) (0.9238, 14.1877) (0.904, 14.1741) (0.8828, 14.16) (0.8638, 14.1475) (0.5591, 13.9478) (0.2306, 13.8007) (-0.1219, 13.7062) knots 0 0 0 0 0.125 0.125 0.125 0.1875 0.1875 0.1875 0.21875 0.21875 0.21875 0.234375 0.234375 0.234375 0.25 0.25 0.25 0.5 0.5 0.5 0.625 0.625 0.625 0.6875 0.6875 0.6875 0.71875 0.71875 0.71875 0.734375 0.734375 0.734375 0.75 0.75 0.75 1 1 1 1
  line L17 (-4.7883, 15.6589) -> (-4.4696, 15.6589)
  line L18 (-4.7883, 15.6589) -> (-4.4696, 15.6589)
  line L19 (-4.5538, 16.0429) -> (-4.7042, 16.0429)
  ellipse E3 centre (-4.5542, 16.343) end of major axis (-4.7666, 16.5554) minor radius 0.3 (-4.5538, 16.0429) -> (-4.254, 16.3427) ccw
  spline S20 degree 3 poles (-4.4696, 15.6589) (-4.4353, 15.659) (-4.4013, 15.6621) (-4.3679, 15.6678) knots 0 0 0 0 1 1 1 1
  spline S21 degree 3 poles (-4.3679, 15.6678) (-4.3538, 15.6714) (-4.343, 15.6747) (-4.3374, 15.6767) (-4.3363, 15.6771) (-4.3355, 15.6774) (-4.3355, 15.6774) (-4.3351, 15.6776) (-4.3349, 15.6777) (-4.3347, 15.6778) (-4.3347, 15.6779) (-4.3346, 15.6779) (-4.3346, 15.6779) (-4.3346, 15.6779) (-4.3346, 15.6779) (-4.3346, 15.6779) (-4.3346, 15.6779) (-4.3346, 15.6779) (-4.3346, 15.6779) (-4.3347, 15.6779) (-4.3347, 15.6779) (-4.3347, 15.678) (-4.3347, 15.678) (-4.3348, 15.678) (-4.3349, 15.678) (-4.3361, 15.6779) (-4.3393, 15.6772) (-4.3666, 15.6713) (-4.4073, 15.6622) (-4.4696, 15.6589) knots 0 0 0 0 0.216458 0.216458 0.250147 0.250147 0.25213 0.25213 0.266562 0.266562 0.270758 0.270758 0.271952 0.271952 0.272738 0.272738 0.27341 0.27341 0.274154 0.274154 0.275353 0.275353 0.277883 0.277883 0.289351 0.289351 0.40678 0.40678 1 1 1 1
  spline S22 degree 3 poles (-4.3679, 15.6678) (-4.3232, 15.6756) (-4.2796, 15.6882) (-4.2022, 15.7204) (-4.168, 15.7387) (-4.1034, 15.782) (-4.0717, 15.8083) (-4.0175, 15.8623) (-3.9933, 15.8919) (-3.9503, 15.9563) (-3.931, 15.9927) (-3.8857, 16.1003) (-3.8704, 16.1769) (-3.87, 16.2585) knots 0.106772 0.106772 0.106772 0.106772 0.25 0.25 0.375 0.375 0.5 0.5 0.625 0.625 0.75 0.75 1 1 1 1
  arc A6 (-3.7192, 14.351) -> (-4.1621, 14.1709) centre (-3.904, 14.1709) ccw
  spline S23 degree 3 poles (-3.4442, 14.6191) (-3.5354, 14.7125) (-3.6453, 14.7727) (-3.7727, 14.7993) (-3.9002, 14.826) (-4.0253, 14.8146) (-4.1459, 14.7656) (-4.2665, 14.7166) (-4.3639, 14.6373) (-4.4367, 14.5293) (-4.5094, 14.4213) (-4.546, 14.3018) (-4.5461, 14.1709) knots 0 0 0 0 0.25 0.25 0.25 0.5 0.5 0.5 0.75 0.75 0.75 1 1 1 1
  spline S24 degree 3 poles (-3.4442, 14.6191) (-3.5354, 14.7125) (-3.6453, 14.7727) (-3.7727, 14.7993) (-3.9002, 14.826) (-4.0253, 14.8146) (-4.1459, 14.7656) (-4.2665, 14.7166) (-4.3639, 14.6373) (-4.4367, 14.5293) (-4.5094, 14.4213) (-4.546, 14.3018) (-4.5461, 14.1709) knots 0 0 0 0 0.25 0.25 0.25 0.5 0.5 0.5 0.75 0.75 0.75 1 1 1 1
  spline S25 degree 3 poles (-4.4696, 15.6589) (-4.3893, 15.6592) (-4.3104, 15.6755) (-4.2022, 15.7204) (-4.168, 15.7387) (-4.1034, 15.782) (-4.0717, 15.8083) (-4.0175, 15.8623) (-3.9933, 15.8919) (-3.9503, 15.9563) (-3.931, 15.9927) (-3.8857, 16.1003) (-3.8704, 16.1769) (-3.87, 16.2585) knots 0 0 0 0 0.25 0.25 0.375 0.375 0.5 0.5 0.625 0.625 0.75 0.75 1 1 1 1
  spline S26 degree 3 poles (-0.7461, 11.4032) (-0.746, 11.3581) (-0.7425, 11.3136) (-0.7354, 11.2697) (-0.7319, 11.2478) (-0.7275, 11.226) (-0.7223, 11.2043) (-0.717, 11.1826) (-0.7112, 11.1622) (-0.7038, 11.1397) (-0.6741, 11.0495) (-0.6298, 10.9659) (-0.572, 10.8905) (-0.5432, 10.8529) (-0.5115, 10.8181) (-0.4771, 10.7861) (-0.4599, 10.7702) (-0.442, 10.7549) (-0.4234, 10.7403) (-0.4048, 10.7258) (-0.3843, 10.7111) (-0.3655, 10.6988) (-0.2904, 10.6496) (-0.2093, 10.6132) (-0.1219, 10.5898) knots 0 0 0 0 0.125 0.125 0.125 0.1875 0.1875 0.1875 0.25 0.25 0.25 0.5 0.5 0.5 0.625 0.625 0.625 0.6875 0.6875 0.6875 0.75 0.75 0.75 1 1 1 1
  line L20 (-0.7461, 12.8928) -> (-0.7461, 11.4032)
  arc A7 (-1.6459, 12.8928) -> (-1.9854, 13.3353) centre (-2.104, 12.8928) ccw
  line L21 (-1.6459, 11.4032) -> (-1.6459, 12.8928)
  spline S27 degree 3 poles (-1.2619, 12.8928) (-1.2619, 12.9378) (-1.2655, 12.9823) (-1.2725, 13.0262) (-1.2761, 13.0482) (-1.2805, 13.07) (-1.2857, 13.0917) (-1.291, 13.1134) (-1.2968, 13.1337) (-1.3042, 13.1563) (-1.3339, 13.2465) (-1.3782, 13.3301) (-1.4359, 13.4054) (-1.4648, 13.4431) (-1.4965, 13.4779) (-1.5309, 13.5098) (-1.5481, 13.5258) (-1.566, 13.5411) (-1.5846, 13.5556) (-1.6032, 13.5702) (-1.6237, 13.5848) (-1.6425, 13.5971) (-1.7175, 13.6463) (-1.7987, 13.6827) (-1.886, 13.7062) knots 0 0 0 0 0.125 0.125 0.125 0.1875 0.1875 0.1875 0.25 0.25 0.25 0.5 0.5 0.5 0.625 0.625 0.625 0.6875 0.6875 0.6875 0.75 0.75 0.75 1 1 1 1
  spline S28 degree 3 poles (-1.2619, 12.8928) (-1.2619, 12.9378) (-1.2655, 12.9823) (-1.2725, 13.0262) (-1.2761, 13.0482) (-1.2805, 13.07) (-1.2857, 13.0917) (-1.291, 13.1134) (-1.2968, 13.1337) (-1.3042, 13.1563) (-1.3339, 13.2465) (-1.3782, 13.3301) (-1.4359, 13.4054) (-1.4648, 13.4431) (-1.4965, 13.4779) (-1.5309, 13.5098) (-1.5481, 13.5258) (-1.566, 13.5411) (-1.5846, 13.5556) (-1.6032, 13.5702) (-1.6237, 13.5848) (-1.6425, 13.5971) (-1.7175, 13.6463) (-1.7987, 13.6827) (-1.886, 13.7062) knots 0 0 0 0 0.125 0.125 0.125 0.1875 0.1875 0.1875 0.25 0.25 0.25 0.5 0.5 0.5 0.625 0.625 0.625 0.6875 0.6875 0.6875 0.75 0.75 0.75 1 1 1 1
  spline S29 degree 3 poles (-1.886, 10.5898) (-1.8425, 10.6015) (-1.8005, 10.6164) (-1.7599, 10.6346) (-1.7396, 10.6436) (-1.7197, 10.6535) (-1.7001, 10.6643) (-1.6805, 10.675) (-1.6623, 10.6858) (-1.6425, 10.6988) (-1.563, 10.7508) (-1.4938, 10.8153) (-1.4359, 10.8905) (-1.407, 10.9282) (-1.3816, 10.9678) (-1.3596, 11.0093) (-1.3486, 11.03) (-1.3385, 11.0513) (-1.3293, 11.073) (-1.3201, 11.0948) (-1.3112, 11.1184) (-1.3042, 11.1397) (-1.2761, 11.2249) (-1.262, 11.3127) (-1.2619, 11.4032) knots 0 0 0 0 0.125 0.125 0.125 0.1875 0.1875 0.1875 0.25 0.25 0.25 0.5 0.5 0.5 0.625 0.625 0.625 0.6875 0.6875 0.6875 0.75 0.75 0.75 1 1 1 1
  line L22 (-1.2619, 11.4032) -> (-1.2619, 12.8928)
  line L23 (-1.2619, 11.4032) -> (-1.2619, 12.8928)
  line L24 (-0.7461, 12.8928) -> (-0.7461, 11.4032)
  spline S30 degree 3 poles (-0.7461, 11.4032) (-0.746, 11.3581) (-0.7425, 11.3136) (-0.7354, 11.2697) (-0.7319, 11.2478) (-0.7275, 11.226) (-0.7223, 11.2043) (-0.717, 11.1826) (-0.7112, 11.1622) (-0.7038, 11.1397) (-0.6741, 11.0495) (-0.6298, 10.9659) (-0.572, 10.8905) (-0.5432, 10.8529) (-0.5115, 10.8181) (-0.4771, 10.7861) (-0.4599, 10.7702) (-0.442, 10.7549) (-0.4234, 10.7403) (-0.4048, 10.7258) (-0.3843, 10.7111) (-0.3655, 10.6988) (-0.2904, 10.6496) (-0.2093, 10.6132) (-0.1219, 10.5898) knots 0 0 0 0 0.125 0.125 0.125 0.1875 0.1875 0.1875 0.25 0.25 0.25 0.5 0.5 0.5 0.625 0.625 0.625 0.6875 0.6875 0.6875 0.75 0.75 0.75 1 1 1 1
  spline S31 degree 3 poles (-0.1219, 13.7062) (-0.1654, 13.6945) (-0.2075, 13.6796) (-0.2481, 13.6614) (-0.2684, 13.6523) (-0.2883, 13.6424) (-0.3079, 13.6317) (-0.3275, 13.621) (-0.3456, 13.6101) (-0.3655, 13.5972) (-0.4449, 13.5452) (-0.5142, 13.4807) (-0.5721, 13.4054) (-0.601, 13.3678) (-0.6264, 13.3282) (-0.6484, 13.2867) (-0.6593, 13.2659) (-0.6695, 13.2447) (-0.6787, 13.2229) (-0.6879, 13.2012) (-0.6968, 13.1776) (-0.7038, 13.1563) (-0.7319, 13.0711) (-0.746, 12.9832) (-0.7461, 12.8928) knots 0 0 0 0 0.125 0.125 0.125 0.1875 0.1875 0.1875 0.25 0.25 0.25 0.5 0.5 0.5 0.625 0.625 0.625 0.6875 0.6875 0.6875 0.75 0.75 0.75 1 1 1 1
  spline S32 degree 3 poles (-0.1219, 13.7062) (-0.1654, 13.6945) (-0.2075, 13.6796) (-0.2481, 13.6614) (-0.2684, 13.6523) (-0.2883, 13.6424) (-0.3079, 13.6317) (-0.3275, 13.621) (-0.3456, 13.6101) (-0.3655, 13.5972) (-0.4449, 13.5452) (-0.5142, 13.4807) (-0.5721, 13.4054) (-0.601, 13.3678) (-0.6264, 13.3282) (-0.6484, 13.2867) (-0.6593, 13.2659) (-0.6695, 13.2447) (-0.6787, 13.2229) (-0.6879, 13.2012) (-0.6968, 13.1776) (-0.7038, 13.1563) (-0.7319, 13.0711) (-0.746, 12.9832) (-0.7461, 12.8928) knots 0 0 0 0 0.125 0.125 0.125 0.1875 0.1875 0.1875 0.25 0.25 0.25 0.5 0.5 0.5 0.625 0.625 0.625 0.6875 0.6875 0.6875 0.75 0.75 0.75 1 1 1 1
  arc A8 (-0.0226, 13.3353) -> (-0.3621, 12.8928) centre (0.096, 12.8928) ccw
  line L25 (-0.3621, 12.8928) -> (-0.3621, 11.4032)
  line L26 (4.1541, 10.998) -> (4.1541, 6.898)
  line L27 (4.5381, 6.898) -> (4.5381, 10.998)
  spline S33 degree 3 poles (4.5381, 10.998) (4.5381, 11.0398) (4.542, 11.0809) (4.5497, 11.1213) (4.5535, 11.1414) (4.5584, 11.1614) (4.5641, 11.1813) (4.5699, 11.2011) (4.576, 11.2191) (4.5843, 11.2402) (4.6175, 11.3243) (4.6668, 11.3992) (4.7308, 11.4632) (4.7628, 11.4952) (4.7973, 11.5234) (4.8345, 11.5478) (4.8531, 11.5601) (4.8723, 11.5713) (4.8922, 11.5816) (4.9121, 11.5919) (4.9345, 11.602) (4.9538, 11.6097) (5.0313, 11.6404) (5.112, 11.6559) (5.196, 11.6559) knots 0 0 0 0 0.125 0.125 0.125 0.1875 0.1875 0.1875 0.25 0.25 0.25 0.5 0.5 0.5 0.625 0.625 0.625 0.6875 0.6875 0.6875 0.75 0.75 0.75 1 1 1 1
  arc A9 (5.196, 12.0399) -> (4.1541, 10.998) centre (5.196, 10.998) ccw
  line L28 (5.196, 11.6559) -> (6.996, 11.6559)
  line L29 (5.196, 12.0399) -> (6.996, 12.0399)
  arc A10 (6.996, 12.0399) -> (7.4541, 12.498) centre (6.996, 12.498) ccw
  spline S34 degree 3 poles (6.996, 11.6559) (7.0495, 11.6559) (7.1021, 11.6609) (7.1538, 11.6707) (7.1796, 11.6757) (7.2052, 11.6818) (7.2306, 11.6892) (7.256, 11.6966) (7.279, 11.7044) (7.306, 11.715) (7.4138, 11.7576) (7.5094, 11.8206) (7.5914, 11.9025) (7.6325, 11.9435) (7.6686, 11.9878) (7.6998, 12.0353) (7.7155, 12.0591) (7.7299, 12.0838) (7.7431, 12.1092) (7.7497, 12.1219) (7.7559, 12.1349) (7.7619, 12.148) (7.7679, 12.1611) (7.774, 12.1756) (7.779, 12.188) (7.8183, 12.2872) (7.838, 12.3906) (7.8381, 12.498) knots 0 0 0 0 0.125 0.125 0.125 0.1875 0.1875 0.1875 0.25 0.25 0.25 0.5 0.5 0.5 0.625 0.625 0.625 0.6875 0.6875 0.6875 0.71875 0.71875 0.71875 0.75 0.75 0.75 1 1 1 1
  spline S35 degree 3 poles (6.996, 11.6559) (7.0495, 11.6559) (7.1021, 11.6609) (7.1538, 11.6707) (7.1796, 11.6757) (7.2052, 11.6818) (7.2306, 11.6892) (7.256, 11.6966) (7.279, 11.7044) (7.306, 11.715) (7.4138, 11.7576) (7.5094, 11.8206) (7.5914, 11.9025) (7.6325, 11.9435) (7.6686, 11.9878) (7.6998, 12.0353) (7.7155, 12.0591) (7.7299, 12.0838) (7.7431, 12.1092) (7.7497, 12.1219) (7.7559, 12.1349) (7.7619, 12.148) (7.7679, 12.1611) (7.774, 12.1756) (7.779, 12.188) (7.8183, 12.2872) (7.838, 12.3906) (7.8381, 12.498) knots 0 0 0 0 0.125 0.125 0.125 0.1875 0.1875 0.1875 0.25 0.25 0.25 0.5 0.5 0.5 0.625 0.625 0.625 0.6875 0.6875 0.6875 0.71875 0.71875 0.71875 0.75 0.75 0.75 1 1 1 1
  line L30 (5.196, 11.6559) -> (6.996, 11.6559)
  spline S36 degree 3 poles (4.5381, 10.998) (4.5381, 11.0398) (4.542, 11.0809) (4.5497, 11.1213) (4.5535, 11.1414) (4.5584, 11.1614) (4.5641, 11.1813) (4.5699, 11.2011) (4.576, 11.2191) (4.5843, 11.2402) (4.6175, 11.3243) (4.6668, 11.3992) (4.7308, 11.4632) (4.7628, 11.4952) (4.7973, 11.5234) (4.8345, 11.5478) (4.8531, 11.5601) (4.8723, 11.5713) (4.8922, 11.5816) (4.9121, 11.5919) (4.9345, 11.602) (4.9538, 11.6097) (5.0313, 11.6404) (5.112, 11.6559) (5.196, 11.6559) knots 0 0 0 0 0.125 0.125 0.125 0.1875 0.1875 0.1875 0.25 0.25 0.25 0.5 0.5 0.5 0.625 0.625 0.625 0.6875 0.6875 0.6875 0.75 0.75 0.75 1 1 1 1
  line L31 (4.5381, 6.898) -> (4.5381, 10.998)
  arc A11 (3.696, 6.4399) -> (4.1541, 6.898) centre (3.696, 6.898) ccw
  line L32 (3.246, 6.4399) -> (3.696, 6.4399)
  line L33 (3.696, 5.1561) -> (3.246, 5.1561)
  line L34 (3.246, 6.0559) -> (3.696, 6.0559)
  line L35 (3.246, 6.0559) -> (3.696, 6.0559)
  line L36 (3.696, 5.5401) -> (3.246, 5.5401)
  line L37 (3.696, 5.5401) -> (3.246, 5.5401)
  arc A12 (4.1541, 4.698) -> (3.696, 5.1561) centre (3.696, 4.698) ccw
  spline S37 degree 3 poles (4.5381, 4.698) (4.5381, 4.7515) (4.533, 4.8041) (4.5232, 4.8558) (4.5183, 4.8816) (4.5121, 4.9072) (4.5048, 4.9326) (4.4974, 4.9579) (4.4896, 4.981) (4.479, 5.0079) (4.4363, 5.1157) (4.3734, 5.2114) (4.2914, 5.2934) (4.2505, 5.3344) (4.2061, 5.3704) (4.1585, 5.4017) (4.1348, 5.4173) (4.1102, 5.4317) (4.0848, 5.445) (4.072, 5.4516) (4.0591, 5.4579) (4.046, 5.4639) (4.0329, 5.4699) (4.0184, 5.476) (4.006, 5.4809) (3.9067, 5.5202) (3.8034, 5.54) (3.696, 5.5401) knots 0 0 0 0 0.125 0.125 0.125 0.1875 0.1875 0.1875 0.25 0.25 0.25 0.5 0.5 0.5 0.625 0.625 0.625 0.6875 0.6875 0.6875 0.71875 0.71875 0.71875 0.75 0.75 0.75 1 1 1 1
  spline S38 degree 3 poles (4.5381, 4.698) (4.5381, 4.7515) (4.533, 4.8041) (4.5232, 4.8558) (4.5183, 4.8816) (4.5121, 4.9072) (4.5048, 4.9326) (4.4974, 4.9579) (4.4896, 4.981) (4.479, 5.0079) (4.4363, 5.1157) (4.3734, 5.2114) (4.2914, 5.2934) (4.2505, 5.3344) (4.2061, 5.3704) (4.1585, 5.4017) (4.1348, 5.4173) (4.1102, 5.4317) (4.0848, 5.445) (4.072, 5.4516) (4.0591, 5.4579) (4.046, 5.4639) (4.0329, 5.4699) (4.0184, 5.476) (4.006, 5.4809) (3.9067, 5.5202) (3.8034, 5.54) (3.696, 5.5401) knots 0 0 0 0 0.125 0.125 0.125 0.1875 0.1875 0.1875 0.25 0.25 0.25 0.5 0.5 0.5 0.625 0.625 0.625 0.6875 0.6875 0.6875 0.71875 0.71875 0.71875 0.75 0.75 0.75 1 1 1 1
  spline S39 degree 3 poles (3.696, 6.0559) (3.7495, 6.0559) (3.8021, 6.0609) (3.8538, 6.0707) (3.8796, 6.0757) (3.9052, 6.0818) (3.9306, 6.0892) (3.956, 6.0966) (3.979, 6.1044) (4.006, 6.115) (4.1138, 6.1576) (4.2094, 6.2206) (4.2914, 6.3025) (4.3325, 6.3435) (4.3686, 6.3878) (4.3998, 6.4353) (4.4155, 6.4591) (4.4299, 6.4838) (4.4431, 6.5092) (4.4497, 6.5219) (4.4559, 6.5349) (4.4619, 6.548) (4.4679, 6.5611) (4.474, 6.5756) (4.479, 6.588) (4.5183, 6.6872) (4.538, 6.7906) (4.5381, 6.898) knots 0 0 0 0 0.125 0.125 0.125 0.1875 0.1875 0.1875 0.25 0.25 0.25 0.5 0.5 0.5 0.625 0.625 0.625 0.6875 0.6875 0.6875 0.71875 0.71875 0.71875 0.75 0.75 0.75 1 1 1 1
  spline S40 degree 3 poles (3.696, 6.0559) (3.7495, 6.0559) (3.8021, 6.0609) (3.8538, 6.0707) (3.8796, 6.0757) (3.9052, 6.0818) (3.9306, 6.0892) (3.956, 6.0966) (3.979, 6.1044) (4.006, 6.115) (4.1138, 6.1576) (4.2094, 6.2206) (4.2914, 6.3025) (4.3325, 6.3435) (4.3686, 6.3878) (4.3998, 6.4353) (4.4155, 6.4591) (4.4299, 6.4838) (4.4431, 6.5092) (4.4497, 6.5219) (4.4559, 6.5349) (4.4619, 6.548) (4.4679, 6.5611) (4.474, 6.5756) (4.479, 6.588) (4.5183, 6.6872) (4.538, 6.7906) (4.5381, 6.898) knots 0 0 0 0 0.125 0.125 0.125 0.1875 0.1875 0.1875 0.25 0.25 0.25 0.5 0.5 0.5 0.625 0.625 0.625 0.6875 0.6875 0.6875 0.71875 0.71875 0.71875 0.75 0.75 0.75 1 1 1 1
  spline S41 degree 3 poles (-0.1219, 10.5898) (0.0541, 10.5426) (0.2243, 10.4822) (0.3886, 10.4086) (0.4707, 10.3719) (0.5514, 10.3318) (0.6306, 10.2884) (0.6702, 10.2667) (0.7094, 10.2442) (0.7483, 10.2209) (0.7677, 10.2093) (0.7871, 10.1974) (0.8063, 10.1853) (0.8256, 10.1732) (0.8436, 10.1617) (0.8638, 10.1485) (1.186, 9.9374) (1.4652, 9.6782) (1.6997, 9.3726) (1.817, 9.2198) (1.92, 9.0594) (2.0089, 8.8913) (2.0533, 8.8073) (2.0942, 8.7214) (2.1315, 8.6335) (2.1502, 8.5896) (2.1679, 8.5452) (2.1848, 8.5004) (2.1933, 8.4779) (2.2015, 8.4554) (2.2095, 8.4327) (2.2175, 8.41) (2.2257, 8.386) (2.2328, 8.3643) (2.3468, 8.0184) (2.4039, 7.6629) (2.4039, 7.298) knots 0 0 0 0 0.125 0.125 0.125 0.1875 0.1875 0.1875 0.21875 0.21875 0.21875 0.234375 0.234375 0.234375 0.25 0.25 0.25 0.5 0.5 0.5 0.625 0.625 0.625 0.6875 0.6875 0.6875 0.71875 0.71875 0.71875 0.734375 0.734375 0.734375 0.75 0.75 0.75 1 1 1 1
  arc A13 (2.7879, 7.298) -> (-0.0226, 10.9607) centre (-1.004, 7.298) ccw
  arc A14 (-0.3621, 11.4032) -> (-0.0226, 10.9607) centre (0.096, 11.4032) ccw
  line L38 (2.4039, 7.298) -> (2.4039, 6.898)
  spline S42 degree 3 poles (-0.1219, 10.5898) (0.0541, 10.5426) (0.2243, 10.4822) (0.3886, 10.4086) (0.4707, 10.3719) (0.5514, 10.3318) (0.6306, 10.2884) (0.6702, 10.2667) (0.7094, 10.2442) (0.7483, 10.2209) (0.7677, 10.2093) (0.7871, 10.1974) (0.8063, 10.1853) (0.8256, 10.1732) (0.8436, 10.1617) (0.8638, 10.1485) (1.186, 9.9374) (1.4652, 9.6782) (1.6997, 9.3726) (1.817, 9.2198) (1.92, 9.0594) (2.0089, 8.8913) (2.0533, 8.8073) (2.0942, 8.7214) (2.1315, 8.6335) (2.1502, 8.5896) (2.1679, 8.5452) (2.1848, 8.5004) (2.1933, 8.4779) (2.2015, 8.4554) (2.2095, 8.4327) (2.2175, 8.41) (2.2257, 8.386) (2.2328, 8.3643) (2.3468, 8.0184) (2.4039, 7.6629) (2.4039, 7.298) knots 0 0 0 0 0.125 0.125 0.125 0.1875 0.1875 0.1875 0.21875 0.21875 0.21875 0.234375 0.234375 0.234375 0.25 0.25 0.25 0.5 0.5 0.5 0.625 0.625 0.625 0.6875 0.6875 0.6875 0.71875 0.71875 0.71875 0.734375 0.734375 0.734375 0.75 0.75 0.75 1 1 1 1
  line L39 (2.4039, 7.298) -> (2.4039, 6.898)
  line L40 (2.7879, 4.298) -> (2.7879, 4.698)
  line L41 (2.7879, 6.898) -> (2.7879, 7.298)
  arc A15 (3.246, 5.1561) -> (2.7879, 4.698) centre (3.246, 4.698) ccw
  spline S43 degree 3 poles (3.246, 5.5401) (3.1925, 5.54) (3.1399, 5.535) (3.0882, 5.5251) (3.0624, 5.5202) (3.0368, 5.5141) (3.0114, 5.5067) (2.9861, 5.4994) (2.963, 5.4916) (2.9361, 5.4809) (2.8283, 5.4383) (2.7326, 5.3753) (2.6506, 5.2934) (2.6096, 5.2524) (2.5736, 5.2081) (2.5423, 5.1605) (2.5189, 5.1248) (2.4981, 5.0874) (2.4801, 5.048) (2.4741, 5.0348) (2.468, 5.0203) (2.4631, 5.0079) (2.4238, 4.9087) (2.404, 4.8054) (2.4039, 4.698) knots 0 0 0 0 0.125 0.125 0.125 0.1875 0.1875 0.1875 0.25 0.25 0.25 0.5 0.5 0.5 0.625 0.625 0.625 0.71875 0.71875 0.71875 0.75 0.75 0.75 1 1 1 1
  spline S44 degree 3 poles (3.246, 5.5401) (3.1925, 5.54) (3.1399, 5.535) (3.0882, 5.5251) (3.0624, 5.5202) (3.0368, 5.5141) (3.0114, 5.5067) (2.9861, 5.4994) (2.963, 5.4916) (2.9361, 5.4809) (2.8283, 5.4383) (2.7326, 5.3753) (2.6506, 5.2934) (2.6096, 5.2524) (2.5736, 5.2081) (2.5423, 5.1605) (2.5189, 5.1248) (2.4981, 5.0874) (2.4801, 5.048) (2.4741, 5.0348) (2.468, 5.0203) (2.4631, 5.0079) (2.4238, 4.9087) (2.404, 4.8054) (2.4039, 4.698) knots 0 0 0 0 0.125 0.125 0.125 0.1875 0.1875 0.1875 0.25 0.25 0.25 0.5 0.5 0.5 0.625 0.625 0.625 0.71875 0.71875 0.71875 0.75 0.75 0.75 1 1 1 1
  spline S45 degree 3 poles (2.4039, 6.898) (2.404, 6.8444) (2.4089, 6.7918) (2.4188, 6.7402) (2.4237, 6.7144) (2.4298, 6.6888) (2.4372, 6.6634) (2.4446, 6.638) (2.4524, 6.615) (2.463, 6.588) (2.5057, 6.4802) (2.5687, 6.3846) (2.6506, 6.3025) (2.6915, 6.2615) (2.7358, 6.2254) (2.7834, 6.1942) (2.8072, 6.1785) (2.8318, 6.1641) (2.8572, 6.1509) (2.8699, 6.1443) (2.8829, 6.1381) (2.896, 6.1321) (2.9092, 6.1261) (2.9236, 6.1199) (2.936, 6.115) (3.0353, 6.0757) (3.1386, 6.056) (3.246, 6.0559) knots 0 0 0 0 0.125 0.125 0.125 0.1875 0.1875 0.1875 0.25 0.25 0.25 0.5 0.5 0.5 0.625 0.625 0.625 0.6875 0.6875 0.6875 0.71875 0.71875 0.71875 0.75 0.75 0.75 1 1 1 1
  spline S46 degree 3 poles (2.4039, 6.898) (2.404, 6.8444) (2.4089, 6.7918) (2.4188, 6.7402) (2.4237, 6.7144) (2.4298, 6.6888) (2.4372, 6.6634) (2.4446, 6.638) (2.4524, 6.615) (2.463, 6.588) (2.5057, 6.4802) (2.5687, 6.3846) (2.6506, 6.3025) (2.6915, 6.2615) (2.7358, 6.2254) (2.7834, 6.1942) (2.8072, 6.1785) (2.8318, 6.1641) (2.8572, 6.1509) (2.8699, 6.1443) (2.8829, 6.1381) (2.896, 6.1321) (2.9092, 6.1261) (2.9236, 6.1199) (2.936, 6.115) (3.0353, 6.0757) (3.1386, 6.056) (3.246, 6.0559) knots 0 0 0 0 0.125 0.125 0.125 0.1875 0.1875 0.1875 0.25 0.25 0.25 0.5 0.5 0.5 0.625 0.625 0.625 0.6875 0.6875 0.6875 0.71875 0.71875 0.71875 0.75 0.75 0.75 1 1 1 1
  arc A16 (2.7879, 6.898) -> (3.246, 6.4399) centre (3.246, 6.898) ccw
  line L42 (-5.388, 8.0375) -> (-5.388, 3.5585)
  line L43 (-5.388, 8.0375) -> (-5.388, 3.5585)
  line L44 (-5.004, 3.6427) -> (-5.004, 7.9533)
  line L45 (-4.254, 7.9533) -> (-4.254, 3.6427)
  line L46 (-3.87, 3.5585) -> (-3.87, 8.0375)
  line L47 (-3.87, 3.5585) -> (-3.87, 8.0375)
  spline S47 degree 3 poles (-4.4696, 2.9589) (-4.3893, 2.9592) (-4.3104, 2.9755) (-4.2022, 3.0204) (-4.168, 3.0387) (-4.1034, 3.082) (-4.0717, 3.1083) (-4.0175, 3.1623) (-3.9933, 3.1919) (-3.9503, 3.2563) (-3.931, 3.2927) (-3.8857, 3.4003) (-3.8704, 3.4769) (-3.87, 3.5585) knots 0 0 0 0 0.25 0.25 0.375 0.375 0.5 0.5 0.625 0.625 0.75 0.75 1 1 1 1